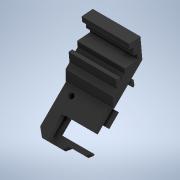
# Autodesk Inventor part: Button Holder
Saved by Autodesk Inventor 2020 (Build 240168000, 168)
## iProperties
Created: 2021-01-14
Part Number: Button Holder
Material: Generic
Document SubType Name: Sheet Metal
Designer: Luke
Density: 1 g/cm^3
Appearance: Default
Sheet Metal Rule: Default
Author: Luke
Autodesk Inventor part; units mm, degrees
ref_plane "Work Plane3" through (59.952259, 18.460087, -23.721288) normal (0, -0.7071068, -0.7071068) x (1, 0, 0)
sketch "Sketch6" plane through (59.952259, 18.460087, -23.721288) normal (0, -0.7071068, -0.7071068) x (1, 0, 0)
  line L0 (-5.715, 11.43) -> (-6.985, 10.16)
  line L1 (-6.985, 10.16) -> (-6.985, -10.16)
  line L2 (-6.985, -10.16) -> (-5.715, -11.43)
  line L3 (-5.715, -11.43) -> (5.715, -11.43)
  line L4 (5.715, 11.43) -> (-5.715, 11.43)
  circle A0 centre (-5.08, 0) radius 0.9525
  line L5 (6.985, 2.5) -> (-4.985, 2.5)
  line L6 (-4.985, -2.5) -> (6.985, -2.5)
  line L7 (6.985, -2.5) -> (6.985, 2.5)
  line L8 (-4.985, -10.02) -> (6.985, -10.02)
  line L9 (6.965, 10.18) -> (-4.985, 10.18)
  line L10 (-4.985, -10.02) -> (-4.985, -2.5)
  line L11 (-4.985, 2.5) -> (-4.985, 10.18)
  line L12 (7.232487, -10.407487) -> (5.859975, -11.78)
  line L13 (5.859975, -11.78) -> (-5.859975, -11.78)
  line L14 (-5.859975, -11.78) -> (-7.335, -10.304975)
  line L15 (-7.335, -10.304975) -> (-7.335, 10.304975)
  line L16 (-7.335, 10.304975) -> (-5.859975, 11.78)
  line L17 (-5.859975, 11.78) -> (5.859975, 11.78)
  line L18 (5.859975, 11.78) -> (7.212487, 10.427487)
  line L19 (6.985, -10.02) -> (6.985, -10.654975)
  line L20 (6.965, 10.18) -> (6.965, 10.674975)
  point P0 (-59.952259, 29.826736)
  point P1 (0, 0)
  dimension "d43" = 0.35
  constraints: 32 end point, 2 perpendicular, 2 point on line, 2 vertical, 1 horizontal, 1 parallel, 4 other
  measures "d43" distance between parallel lines of L3 L13
extrude "Extrusion5" add sketch "Sketch6" along normal blind 2
ref_plane "Work Plane5" through (59.952259, 19.329829, -22.851547) normal (0, 0.7071068, 0.7071068) x (-1, 0, 0)
sketch "Sketch7" plane through (59.952259, 19.329829, -22.851547) normal (0, 0.7071068, 0.7071068) x (-1, 0, 0)
  line L0 (4.985, 10.18) -> (-6.965, 10.18)
  line L1 (-6.965, 10.18) -> (-6.965, 10.674975)
  line L2 (-6.965, 10.674975) -> (-5.859975, 11.78)
  line L3 (-5.859975, 11.78) -> (5.859975, 11.78)
  line L4 (5.859975, 11.78) -> (7.335, 10.304975)
  line L5 (7.335, 10.304975) -> (7.335, -10.304975)
  line L6 (7.335, -10.304975) -> (5.859975, -11.78)
  line L7 (5.859975, -11.78) -> (-5.859975, -11.78)
  line L8 (-5.859975, -11.78) -> (-6.985, -10.654975)
  line L9 (-6.985, -10.654975) -> (-6.985, -10.02)
  line L10 (-6.985, -10.02) -> (4.985, -10.02)
  line L11 (4.985, -10.02) -> (4.985, -2.5)
  line L12 (4.985, -2.5) -> (-6.985, -2.5)
  line L13 (-6.985, -2.5) -> (-6.985, 2.5)
  line L14 (-6.985, 2.5) -> (4.985, 2.5)
  line L15 (4.985, 2.5) -> (4.985, 10.18)
  circle A0 centre (5.08, 0) radius 0.9525
  line L16 (4.985, -2.5) -> (-6.985, -2.5)
  line L17 (4.985, -2.5) -> (-6.985, -2.5)
  line L18 (-6.985, -2.5) -> (-6.985, -5.25)
  line L19 (-6.985, -5.25) -> (4.985, -5.25)
  line L20 (4.985, -5.25) -> (4.985, -2.5)
  line L21 (4.985, 2.5) -> (-6.985, 2.5)
  line L22 (-6.985, 2.5) -> (-6.985, 5.25)
  line L23 (-6.985, 5.25) -> (4.985, 5.25)
  line L24 (4.985, 5.25) -> (4.985, 2.5)
  line L25 (4.985, -10.02) -> (4.985, -2.5)
  line L26 (4.985, -10.02) -> (-6.985, -10.02)
  line L27 (-6.985, -10.02) -> (-6.985, -7.29)
  line L28 (-6.985, -7.29) -> (4.985, -7.29)
  line L29 (4.985, -7.29) -> (4.985, -10.02)
  line L30 (4.985, 10.18) -> (4.985, 11.78)
  line L31 (-5.859975, 11.78) -> (5.859975, 11.78)
  point P0 (4.985, 5.25)
  point P1 (4.985, -7.29)
  point P2 (4.985, 11.78)
  dimension "d67" = 11.97
  dimension "d68" = 2.75
  dimension "d69" = 2.75
  constraints: 26 end point, 6 parallel, 4 perpendicular, 3 horizontal, 1 point on line
  measures "d67" distance of L19.end L18.end
  measures "d68" distance of L18.end L17.end
  measures "d69" distance of L21.end L22.end
extrude "Extrusion6" add sketch "Sketch7" along normal blind 2 contours L30 L3 L4 L5 L6 L7 L8 L9 L10 L11 L12 L13 L14 L15 | L15 L14 L22 L23 | L12 L11 L19 L18 | L11 L10 L27 L28
sketch "Sketch8" plane through (66.937259, 16.69232, -21.953521) normal (1, 0, 0) x (0, -0.7071068, -0.7071068)
  line L0 (0, 3.4525) -> (0, 1.5475)
  line L1 (0, 2.5) -> (-1.23, 2.5)
  line L2 (-1.23, 1.5475) -> (-1.23, 3.4525)
  line L3 (-1.315, 16.564694) -> (0.085, 16.564694)
  line L4 (0.085, 16.564694) -> (0.085, -11.564694)
  line L5 (0.085, -11.564694) -> (-1.315, -11.564694)
  line L6 (-1.315, -11.564694) -> (-1.315, 16.564694)
  line L7 (-1.315, 16.564694) -> (0.085, -11.564694) construction
  line L8 (0.085, 16.564694) -> (-1.315, -11.564694) construction
  point P0 (-3.720231, -27.326736)
  point P1 (-0.615, 2.5)
  dimension "d48" = 1.4
  constraints: 14 end point, 5 midpoint, 2 parallel, 1 horizontal, 1 perpendicular
  measures "d48" distance of L4.end L5.end
extrude "Extrusion7" cut sketch "Sketch8" against normal through all
sketch "Sketch9" plane through (59.952259, 17.045874, -25.135502) normal (0, -0.7071068, -0.7071068) x (-1, 0, 0)
  line L0 (0, -11.78) -> (5.859975, -11.78)
  line L1 (5.859975, -11.78) -> (7.335, -10.304975)
  line L2 (7.335, -10.304975) -> (7.335, 10.304975)
  line L3 (7.335, 10.304975) -> (5.859975, 11.78)
  line L4 (5.859975, 11.78) -> (0, 11.78)
  line L5 (1.5, 13.28) -> (6.481295, 13.28)
  line L6 (6.481295, 13.28) -> (8.835, 10.926295)
  line L7 (8.835, 10.926295) -> (8.835, -10.926295)
  line L8 (8.835, -10.926295) -> (6.481295, -13.28)
  line L9 (6.481295, -13.28) -> (1.5, -13.28)
  line L10 (-5.859975, -11.78) -> (5.859975, -11.78)
  line L11 (0, 11.78) -> (1.5, 13.28)
  line L12 (0, 11.78) -> (2.12132, 11.78) construction
  line L13 (0, -11.78) -> (1.5, -13.28)
  line L14 (0, -11.78) -> (2.12132, -11.78) construction
  point P0 (4.985, -10.18)
  dimension "d215" = 1.78
  dimension "d51" = 1.5
  dimension "d65" = 45
  dimension "d66" = 45
  constraints: 22 end point, 2 equal length, 2 horizontal, 2 other
  measures "d51" distance between parallel lines of L4 L5
  measures "d65" angle of L12 L11
  measures "d66" angle of L13 L14
extrude "Extrusion8" add sketch "Sketch9" against normal up to surface (5.23 mm away)
sketch "Sketch10" plane through (59.952259, 20.744042, -21.437333) normal (0, 0.7071068, 0.7071068) x (1, 0, 0)
  line L0 (-1.5, -13.28) -> (-4.985, -13.28)
  line L1 (0, -11.78) -> (-1.5, -13.28)
  line L2 (-4.985, -11.78) -> (0, -11.78)
  line L3 (-4.985, -11.78) -> (0, -11.78) projected
  line L4 (-4.985, -11.78) -> (-4.985, -13.28)
  constraints: 8 end point, 1 perpendicular
extrude "Extrusion9" cut sketch "Sketch10" against normal up to surface (3.315 mm away)
ref_plane "Work Plane6" through (29.805274, 44.348366, 88.772132) normal (1, 0, 0) x (0, 1, 0)
ref_plane "Work Plane12" through (54.967259, 17.045874, -25.135502) normal (0, -0.7071068, 0.7071068) x (1, 0, 0)
ref_plane "Work Plane17" through (68.724834, 47.176122, -18.749118) normal (1, 0, 0) x (0, 0, -1)
sketch "Sketch20" plane through (68.724834, 47.176122, -18.749118) normal (1, 0, 0) x (0, 0, -1)
  line L0 (13.419594, -13.20803) -> (8.638979, -13.62628)
  line L1 (15.035179, -14.09038) -> (14.351109, -6.271416)
  line L2 (14.351109, -6.271416) -> (10.333918, -6.622875)
  line L3 (10.333918, -6.622875) -> (10.490847, -8.41658)
  line L4 (10.490847, -8.41658) -> (11.736127, -8.307632)
  line L5 (11.736127, -8.307632) -> (11.982597, -11.124789)
  line L6 (11.982597, -11.124789) -> (13.227803, -11.015847)
  line L7 (13.227803, -11.015847) -> (13.419594, -13.20803)
  line L8 (2.423047, -22.458344) -> (4.545131, -24.580428)
  line L9 (15.035179, -14.09038) -> (4.545131, -24.580428)
  line L10 (2.139996, -15.701569) -> (8.620368, -15.13461)
  line L11 (8.620368, -15.13461) -> (8.164544, -9.924512)
  line L12 (8.822224, -15.72077) -> (8.638979, -13.62628)
  line L13 (7.051339, -17.279522) -> (6.877028, -15.287133)
  line L14 (6.929946, -17.613048) -> (6.740672, -15.449635)
  line L15 (6.740672, -15.449635) -> (5.495428, -15.55858)
  line L16 (6.740672, -15.449635) -> (7.990672, -15.449635) construction
  line L17 (5.495428, -15.55858) -> (5.803342, -19.078049)
  line L18 (5.803342, -19.078049) -> (2.423047, -22.458344)
  line L19 (8.666698, -15.664163) -> (7.051339, -17.279522)
  line L20 (6.929946, -17.613048) -> (8.822224, -15.72077)
  point P0 (9.190892, -19.934667)
  dimension "d239" = 1.25
  dimension "d240" = 175
  dimension "d241" = 90
  constraints: 42 end point, 1 equal length, 1 horizontal, 1 point on line, 10 other
  measures "d239" distance of L14.end L15.end
  measures "d240" angle of L15 L16
  measures "d241" angle of L17 L15
extrude "Extrusion13" add sketch "Sketch20" against normal up to surface (17.607575 mm away)
ref_plane "Work Plane23" through (59.921046, 47.176122, -18.749118) normal (1, 0, 0) x (0, 0, -1)
chamfer "Chamfer7" distance 1.78 angle 45 7 edges at (62.8822, 29.0711, -29.7697) (59.2023, 29.6015, -30.3) (66.9373, 27.0859, -27.7845) (66.3747, 28.6734, -29.3719) (55.9616, 30.1318, -30.8303) (52.2941, 29.2996, -29.9982) (66.9373, 23.5247, -24.2233)
chamfer "Chamfer8" distance 2.75 angle 45 1 edges at (59.921, 24.7178, -21.1722)
body "Solid1"
